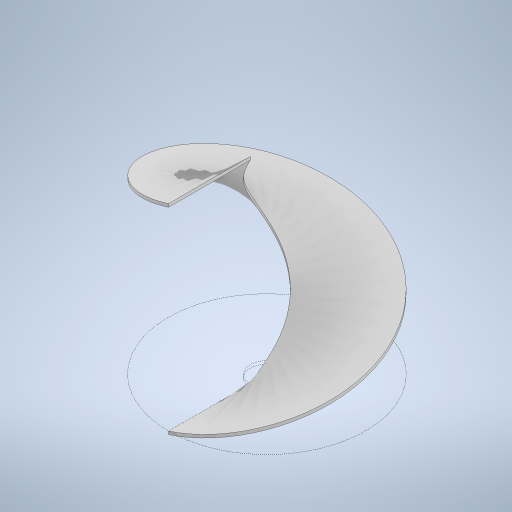
# Autodesk Inventor part: Espira_01
Saved by Autodesk Inventor 2024 (Build 280153000, 153)
## iProperties
Created: 2026-01-07
Part Number: Espira_01
Material: Generic
Document SubType Name: Modeling
Designer: eduso
Density: 1 g/cm^3
Appearance: Default
Paso_Espira_01: 200,000 mm
ø_Ext_Espira_01: 200,000 mm
ø_Int_Espira_01: 33,700 mm
Espesor_Espira_01: 3,200 mm
Author: eduso
Autodesk Inventor part; units mm, degrees
ref_plane "YZ Plane" through (0, 0, 0) normal (1, 0, 0) x (0, 1, 0)
ref_plane "XY Plane" through (0, 0, 0) normal (0, 0, 1) x (1, 0, 0)
sketch "Sketch1" plane through (0, 0, 0) normal (0, 1, 0) x (-1, 0, 0)
  circle A0 centre (0, 0) radius 16.85 construction
  line L0 (0, 0) -> (0, 16.85) construction
  dimension "d0" = 33.7
  constraints: 2 end point, 1 coincident, 1 vertical, 1 vertical alignment, 2 other
ref_plane "Work Plane1" through (0, 3.2, 0) normal (0, 1, 0) x (-1, 0, 0)
sketch "Sketch2" plane through (0, 3.2, 0) normal (0, 1, 0) x (-1, 0, 0)
  circle A0 centre (0, 0) radius 100 construction
  line L0 (0, 0) -> (0, 100) construction
  circle A1 centre (0, 0) radius 16.85 construction
  dimension "d2" = 200
  dimension "d12" = 33.7
  constraints: 2 coincident, 2 end point, 1 centre point, 1 vertical, 1 vertical alignment, 2 other
  measures "d12" diameter of A1
sketch "Sketch3" plane through (0, 0, 0) normal (1, 0, 0) x (0, 1, 0)
  line L0 (0, 0) -> (200, 0) construction
  line L1 (0, 16.85) -> (3.2, 16.85)
  line L2 (3.2, 16.85) -> (3.2, 100)
  line L3 (3.2, 100) -> (0, 100)
  line L4 (0, 100) -> (0, 16.85)
  dimension "d3" = 200
  dimension "d13" = 16.85
  dimension "d14" = 100
  dimension "d15" = 3.2
  constraints: 10 end point, 2 horizontal, 2 parallel, 1 perpendicular
  measures "d3" distance of L0.start L0.end
  measures "d13" distance between parallel lines of L0 L1
  measures "d14" distance between parallel lines of L0 L3
  measures "d15" distance of L1.start L1.end
coil "Coil1" sketch "Sketch3" operation add axis through (0, 0, 0) along (0, 1, 0) pitch 200 turns 1 hand right
equation "\"d0\" = ø_Int_Espira_01"
equation "\"d2\" = ø_Ext_Espira_01"
equation "\"d12\" = ø_Int_Espira_01"
equation "\"d13\" = 0.5 * ø_Int_Espira_01"
equation "\"d14\" = 0.5 * ø_Ext_Espira_01"
equation "\"d15\" = Espesor_Espira_01"
equation "\"ø_Ext_Espira_01\" = 200"
equation "\"ø_Int_Espira_01\" = 33.7"
equation "\"Espesor_Espira_01\" = 3.2"
equation "\"d1\" = Espesor_Espira_01"
body "Solid1"
